Autodesk Inventor part; units mm, degrees
(part 2 of 2)
  arc A318 (-2.0424, 4.8628) -> (-1.7451, 4.6028) centre (-1.7451, 4.9028) ccw
  arc A319 (-4.2549, 4.6028) -> (-3.9576, 4.8628) centre (-4.2549, 4.9028) ccw
  line L244 (-4.5, 4.6028) -> (-4.2549, 4.6028)
  line L245 (-1.7451, 4.6028) -> (-1.5, 4.6028)
  arc A320 (-2.0424, 4.8628) -> (-2.4783, 5.8528) centre (-3.975, 4.6028) ccw
  line L246 (-3.5217, 5.8528) -> (-2.4783, 5.8528)
  arc A321 (-3.5217, 5.8528) -> (-3.9576, 4.8628) centre (-2.025, 4.6028) ccw
  arc A322 (-5.0424, 4.8628) -> (-4.7451, 4.6028) centre (-4.7451, 4.9028) ccw
  arc A323 (-7.2549, 4.6028) -> (-6.9576, 4.8628) centre (-7.2549, 4.9028) ccw
  line L247 (-7.5, 4.6028) -> (-7.2549, 4.6028)
  line L248 (-4.7451, 4.6028) -> (-4.5, 4.6028)
  arc A324 (-5.0424, 4.8628) -> (-5.4783, 5.8528) centre (-6.975, 4.6028) ccw
  line L249 (-6.5217, 5.8528) -> (-5.4783, 5.8528)
  arc A325 (-6.5217, 5.8528) -> (-6.9576, 4.8628) centre (-5.025, 4.6028) ccw
  arc A326 (24.9576, 4.8628) -> (25.2549, 4.6028) centre (25.2549, 4.9028) ccw
  arc A327 (22.7451, 4.6028) -> (23.0424, 4.8628) centre (22.7451, 4.9028) ccw
  line L250 (22.5, 4.6028) -> (22.7451, 4.6028)
  line L251 (25.2549, 4.6028) -> (25.5, 4.6028)
  arc A328 (24.9576, 4.8628) -> (24.5217, 5.8528) centre (23.025, 4.6028) ccw
  line L252 (23.4783, 5.8528) -> (24.5217, 5.8528)
  arc A329 (23.4783, 5.8528) -> (23.0424, 4.8628) centre (24.975, 4.6028) ccw
  arc A330 (21.9576, 4.8628) -> (22.2549, 4.6028) centre (22.2549, 4.9028) ccw
  arc A331 (19.7451, 4.6028) -> (20.0424, 4.8628) centre (19.7451, 4.9028) ccw
  line L253 (19.5, 4.6028) -> (19.7451, 4.6028)
  line L254 (22.2549, 4.6028) -> (22.5, 4.6028)
  arc A332 (21.9576, 4.8628) -> (21.5217, 5.8528) centre (20.025, 4.6028) ccw
  line L255 (20.4783, 5.8528) -> (21.5217, 5.8528)
  arc A333 (20.4783, 5.8528) -> (20.0424, 4.8628) centre (21.975, 4.6028) ccw
  arc A334 (18.9576, 4.8628) -> (19.2549, 4.6028) centre (19.2549, 4.9028) ccw
  arc A335 (16.7451, 4.6028) -> (17.0424, 4.8628) centre (16.7451, 4.9028) ccw
  line L256 (16.5, 4.6028) -> (16.7451, 4.6028)
  line L257 (19.2549, 4.6028) -> (19.5, 4.6028)
  arc A336 (18.9576, 4.8628) -> (18.5217, 5.8528) centre (17.025, 4.6028) ccw
  line L258 (17.4783, 5.8528) -> (18.5217, 5.8528)
  arc A337 (17.4783, 5.8528) -> (17.0424, 4.8628) centre (18.975, 4.6028) ccw
  arc A338 (15.9576, 4.8628) -> (16.2549, 4.6028) centre (16.2549, 4.9028) ccw
  arc A339 (13.7451, 4.6028) -> (14.0424, 4.8628) centre (13.7451, 4.9028) ccw
  line L259 (13.5, 4.6028) -> (13.7451, 4.6028)
  line L260 (16.2549, 4.6028) -> (16.5, 4.6028)
  arc A340 (15.9576, 4.8628) -> (15.5217, 5.8528) centre (14.025, 4.6028) ccw
  line L261 (14.4783, 5.8528) -> (15.5217, 5.8528)
  arc A341 (14.4783, 5.8528) -> (14.0424, 4.8628) centre (15.975, 4.6028) ccw
  arc A342 (12.9576, 4.8628) -> (13.2549, 4.6028) centre (13.2549, 4.9028) ccw
  arc A343 (10.7451, 4.6028) -> (11.0424, 4.8628) centre (10.7451, 4.9028) ccw
  line L262 (10.5, 4.6028) -> (10.7451, 4.6028)
  line L263 (13.2549, 4.6028) -> (13.5, 4.6028)
  arc A344 (12.9576, 4.8628) -> (12.5217, 5.8528) centre (11.025, 4.6028) ccw
  line L264 (11.4783, 5.8528) -> (12.5217, 5.8528)
  arc A345 (11.4783, 5.8528) -> (11.0424, 4.8628) centre (12.975, 4.6028) ccw
  arc A346 (9.9576, 4.8628) -> (10.2549, 4.6028) centre (10.2549, 4.9028) ccw
  arc A347 (7.7451, 4.6028) -> (8.0424, 4.8628) centre (7.7451, 4.9028) ccw
  line L265 (7.5, 4.6028) -> (7.7451, 4.6028)
  line L266 (10.2549, 4.6028) -> (10.5, 4.6028)
  arc A348 (9.9576, 4.8628) -> (9.5217, 5.8528) centre (8.025, 4.6028) ccw
  line L267 (8.4783, 5.8528) -> (9.5217, 5.8528)
  arc A349 (8.4783, 5.8528) -> (8.0424, 4.8628) centre (9.975, 4.6028) ccw
  arc A350 (6.9576, 4.8628) -> (7.2549, 4.6028) centre (7.2549, 4.9028) ccw
  arc A351 (4.7451, 4.6028) -> (5.0424, 4.8628) centre (4.7451, 4.9028) ccw
  line L268 (4.5, 4.6028) -> (4.7451, 4.6028)
  line L269 (7.2549, 4.6028) -> (7.5, 4.6028)
  arc A352 (6.9576, 4.8628) -> (6.5217, 5.8528) centre (5.025, 4.6028) ccw
  line L270 (5.4783, 5.8528) -> (6.5217, 5.8528)
  arc A353 (5.4783, 5.8528) -> (5.0424, 4.8628) centre (6.975, 4.6028) ccw
  arc A354 (3.9576, 4.8628) -> (4.2549, 4.6028) centre (4.2549, 4.9028) ccw
  arc A355 (1.7451, 4.6028) -> (2.0424, 4.8628) centre (1.7451, 4.9028) ccw
  line L271 (1.5, 4.6028) -> (1.7451, 4.6028)
  line L272 (4.2549, 4.6028) -> (4.5, 4.6028)
  arc A356 (3.9576, 4.8628) -> (3.5217, 5.8528) centre (2.025, 4.6028) ccw
  line L273 (2.4783, 5.8528) -> (3.5217, 5.8528)
  arc A357 (2.4783, 5.8528) -> (2.0424, 4.8628) centre (3.975, 4.6028) ccw
  arc A358 (0.9576, 4.8628) -> (1.2549, 4.6028) centre (1.2549, 4.9028) ccw
  arc A359 (-1.2549, 4.6028) -> (-0.9576, 4.8628) centre (-1.2549, 4.9028) ccw
  line L274 (-1.5, 4.6028) -> (-1.2549, 4.6028)
  line L275 (1.2549, 4.6028) -> (1.5, 4.6028)
  arc A360 (0.9576, 4.8628) -> (0.5217, 5.8528) centre (-0.975, 4.6028) ccw
  line L276 (-0.5217, 5.8528) -> (0.5217, 5.8528)
  arc A361 (-0.5217, 5.8528) -> (-0.9576, 4.8628) centre (0.975, 4.6028) ccw
  arc A362 (-2.0424, 4.8628) -> (-1.7451, 4.6028) centre (-1.7451, 4.9028) ccw
  arc A363 (-4.2549, 4.6028) -> (-3.9576, 4.8628) centre (-4.2549, 4.9028) ccw
  line L277 (-4.5, 4.6028) -> (-4.2549, 4.6028)
  line L278 (-1.7451, 4.6028) -> (-1.5, 4.6028)
  arc A364 (-2.0424, 4.8628) -> (-2.4783, 5.8528) centre (-3.975, 4.6028) ccw
  line L279 (-3.5217, 5.8528) -> (-2.4783, 5.8528)
  arc A365 (-3.5217, 5.8528) -> (-3.9576, 4.8628) centre (-2.025, 4.6028) ccw
  arc A366 (27.9576, 4.8628) -> (28.2549, 4.6028) centre (28.2549, 4.9028) ccw
  arc A367 (25.7451, 4.6028) -> (26.0424, 4.8628) centre (25.7451, 4.9028) ccw
  line L280 (25.5, 4.6028) -> (25.7451, 4.6028)
  line L281 (28.2549, 4.6028) -> (28.5, 4.6028)
  arc A368 (27.9576, 4.8628) -> (27.5217, 5.8528) centre (26.025, 4.6028) ccw
  line L282 (26.4783, 5.8528) -> (27.5217, 5.8528)
  arc A369 (26.4783, 5.8528) -> (26.0424, 4.8628) centre (27.975, 4.6028) ccw
  arc A370 (24.9576, 4.8628) -> (25.2549, 4.6028) centre (25.2549, 4.9028) ccw
  arc A371 (22.7451, 4.6028) -> (23.0424, 4.8628) centre (22.7451, 4.9028) ccw
  line L283 (22.5, 4.6028) -> (22.7451, 4.6028)
  line L284 (25.2549, 4.6028) -> (25.5, 4.6028)
  arc A372 (24.9576, 4.8628) -> (24.5217, 5.8528) centre (23.025, 4.6028) ccw
  line L285 (23.4783, 5.8528) -> (24.5217, 5.8528)
  arc A373 (23.4783, 5.8528) -> (23.0424, 4.8628) centre (24.975, 4.6028) ccw
  arc A374 (21.9576, 4.8628) -> (22.2549, 4.6028) centre (22.2549, 4.9028) ccw
  arc A375 (19.7451, 4.6028) -> (20.0424, 4.8628) centre (19.7451, 4.9028) ccw
  line L286 (19.5, 4.6028) -> (19.7451, 4.6028)
  line L287 (22.2549, 4.6028) -> (22.5, 4.6028)
  arc A376 (21.9576, 4.8628) -> (21.5217, 5.8528) centre (20.025, 4.6028) ccw
  line L288 (20.4783, 5.8528) -> (21.5217, 5.8528)
  arc A377 (20.4783, 5.8528) -> (20.0424, 4.8628) centre (21.975, 4.6028) ccw
  arc A378 (18.9576, 4.8628) -> (19.2549, 4.6028) centre (19.2549, 4.9028) ccw
  arc A379 (16.7451, 4.6028) -> (17.0424, 4.8628) centre (16.7451, 4.9028) ccw
  line L289 (16.5, 4.6028) -> (16.7451, 4.6028)
  line L290 (19.2549, 4.6028) -> (19.5, 4.6028)
  arc A380 (18.9576, 4.8628) -> (18.5217, 5.8528) centre (17.025, 4.6028) ccw
  line L291 (17.4783, 5.8528) -> (18.5217, 5.8528)
  arc A381 (17.4783, 5.8528) -> (17.0424, 4.8628) centre (18.975, 4.6028) ccw
  arc A382 (15.9576, 4.8628) -> (16.2549, 4.6028) centre (16.2549, 4.9028) ccw
  arc A383 (13.7451, 4.6028) -> (14.0424, 4.8628) centre (13.7451, 4.9028) ccw
  line L292 (13.5, 4.6028) -> (13.7451, 4.6028)
  line L293 (16.2549, 4.6028) -> (16.5, 4.6028)
  arc A384 (15.9576, 4.8628) -> (15.5217, 5.8528) centre (14.025, 4.6028) ccw
  line L294 (14.4783, 5.8528) -> (15.5217, 5.8528)
  arc A385 (14.4783, 5.8528) -> (14.0424, 4.8628) centre (15.975, 4.6028) ccw
  arc A386 (12.9576, 4.8628) -> (13.2549, 4.6028) centre (13.2549, 4.9028) ccw
  arc A387 (10.7451, 4.6028) -> (11.0424, 4.8628) centre (10.7451, 4.9028) ccw
  line L295 (10.5, 4.6028) -> (10.7451, 4.6028)
  line L296 (13.2549, 4.6028) -> (13.5, 4.6028)
  arc A388 (12.9576, 4.8628) -> (12.5217, 5.8528) centre (11.025, 4.6028) ccw
  line L297 (11.4783, 5.8528) -> (12.5217, 5.8528)
  arc A389 (11.4783, 5.8528) -> (11.0424, 4.8628) centre (12.975, 4.6028) ccw
  arc A390 (9.9576, 4.8628) -> (10.2549, 4.6028) centre (10.2549, 4.9028) ccw
  arc A391 (7.7451, 4.6028) -> (8.0424, 4.8628) centre (7.7451, 4.9028) ccw
  line L298 (7.5, 4.6028) -> (7.7451, 4.6028)
  line L299 (10.2549, 4.6028) -> (10.5, 4.6028)
  arc A392 (9.9576, 4.8628) -> (9.5217, 5.8528) centre (8.025, 4.6028) ccw
  line L300 (8.4783, 5.8528) -> (9.5217, 5.8528)
  arc A393 (8.4783, 5.8528) -> (8.0424, 4.8628) centre (9.975, 4.6028) ccw
  arc A394 (6.9576, 4.8628) -> (7.2549, 4.6028) centre (7.2549, 4.9028) ccw
  arc A395 (4.7451, 4.6028) -> (5.0424, 4.8628) centre (4.7451, 4.9028) ccw
  line L301 (4.5, 4.6028) -> (4.7451, 4.6028)
  line L302 (7.2549, 4.6028) -> (7.5, 4.6028)
  arc A396 (6.9576, 4.8628) -> (6.5217, 5.8528) centre (5.025, 4.6028) ccw
  line L303 (5.4783, 5.8528) -> (6.5217, 5.8528)
  arc A397 (5.4783, 5.8528) -> (5.0424, 4.8628) centre (6.975, 4.6028) ccw
  arc A398 (3.9576, 4.8628) -> (4.2549, 4.6028) centre (4.2549, 4.9028) ccw
  arc A399 (1.7451, 4.6028) -> (2.0424, 4.8628) centre (1.7451, 4.9028) ccw
  line L304 (1.5, 4.6028) -> (1.7451, 4.6028)
  line L305 (4.2549, 4.6028) -> (4.5, 4.6028)
  arc A400 (3.9576, 4.8628) -> (3.5217, 5.8528) centre (2.025, 4.6028) ccw
  line L306 (2.4783, 5.8528) -> (3.5217, 5.8528)
  arc A401 (2.4783, 5.8528) -> (2.0424, 4.8628) centre (3.975, 4.6028) ccw
  arc A402 (0.9576, 4.8628) -> (1.2549, 4.6028) centre (1.2549, 4.9028) ccw
  arc A403 (-1.2549, 4.6028) -> (-0.9576, 4.8628) centre (-1.2549, 4.9028) ccw
  line L307 (-1.5, 4.6028) -> (-1.2549, 4.6028)
  line L308 (1.2549, 4.6028) -> (1.5, 4.6028)
  arc A404 (0.9576, 4.8628) -> (0.5217, 5.8528) centre (-0.975, 4.6028) ccw
  line L309 (-0.5217, 5.8528) -> (0.5217, 5.8528)
  arc A405 (-0.5217, 5.8528) -> (-0.9576, 4.8628) centre (0.975, 4.6028) ccw
  point P0 (0, -10)
  point P1 (0, 0)
  point P2 (-0.5217, 5.8528)
  point P3 (-25, 5.8528)
  point P4 (25, 5.8528)
  point P5 (25, 4.7446)
  point P6 (-25, 4.7446)
  dimension "d6" = 16.2338
  dimension "d8" = 100
  dimension "d9" = 0.419
  dimension "d10" = 0.8
  dimension "d12" = 0.3
  dimension "d13" = 0.525
  dimension "d14" = 0.3
  dimension "d15" = 1.95
  dimension "d16" = 2.475
  dimension "d17" = 0.9783
  dimension "d19" = 1.0433
  dimension "d21" = 10
  dimension "d22" = 0.2451
  dimension "d23" = 0.2451
  dimension "d24" = 0.3
  dimension "d25" = 2.7549
  dimension "d26" = 1.25
  dimension "d29" = 0.5217
  dimension "d54" = 3
  dimension "d57" = 3
  constraints: 812 point on circle, 616 end point, 406 centre point, 6 horizontal alignment, 5 tangent, 3 horizontal, 3 parallel, 1 midpoint, 1 point on line, 1 vertical alignment, 1887 other
  measures "d6" radius of A0
  measures "d8" distance of L0.start L0.end
  measures "d9" radial gap between concentric circles of A3 A0
  measures "d10" radial gap between concentric circles of A3 A5
  measures "d12" distance from line of L7 A6.centre
  measures "d13" distance of L7.start A8.centre
  measures "d14" radius of A6
  measures "d15" radius of A7
  measures "d16" distance of L7.start A7.centre
  measures "d17" horizontal distance of L7.start L8.start
  measures "d19" distance of L8.start L8.end
  measures "d21" distance of point (0, 0) point (0, -10)
  measures "d22" distance of L7.start L7.end
  measures "d23" distance of L9.start L9.end
  measures "d24" radius of A9
  measures "d25" distance of L7.start L9.start
  measures "d26" distance from line of L7.start L8
  measures "d29" horizontal distance of point (0, 0) L8.end
  measures "d54" distance of A8.start A10.start
  measures "d57" distance of A8.start A46.start
extrude "押し出し2" cut sketch "スケッチ2" against normal through all contours L10 L11 L12 L3 | L3 L12 A326 A328 L252 A329 A327 L250 L221 A286 A288 L222 A289 A287 L220 L191 A246 A248 L192 A249 A247 L190 L161 A206 A208 L162 A209 A207 L160 L131 A166 A168 L132 A169 A167 L130 L101 A126 A128 L102 A129 A127 L100 L71 A86 A88 L72 A89 A87 L70 L41 A46 A48 L42 A49 A47 L40 L9 A9 A8 L8 A7 A6 L7 L14 A10 A12 L15 A13 A11 L13 L17 A14 A16 L18 A17 A15 L16 L20 A18 A20 L21 A21 A19 L19 L23 A22 A24 L24 A25 A23 L22 L26 A26 A28 L27 A29 A27 L25 L29 A30 A32 L30 A33 A31 L28 L32 A34 A36 L33 A37 A35 L31 L35 A38 A40 L36 A41 A39 L10
sketch "スケッチ6" plane through (0, 0, 8) normal (0, 0, 1) x (1, 0, 0)
  line L0 (-25, -9) -> (25, -9) projected
  line L1 (-25, 4.7446) -> (-25, -9) projected
  line L2 (-25, -9) -> (25, -9)
  line L3 (25, -9) -> (25, 6.6528)
  line L4 (25, 6.6528) -> (-25, 6.6528)
  line L5 (-25, 6.6528) -> (-25, -9)
  line L6 (-23.4783, 5.8528) -> (-24.5217, 5.8528) projected
  point P0 (0, 0)
  dimension "d61" = 0.8
  constraints: 8 end point, 2 parallel, 1 horizontal, 1 perpendicular, 1 vertical alignment
  measures "d61" distance between parallel lines of L4 L6
extrude "押し出し4" add sketch "スケッチ6" along normal blind 8
sketch "スケッチ3" plane through (0, 0, 0) normal (0, 0, 1) x (1, 0, 0)
  point P0 (0, 0)
  point P1 (-15, 0)
  point P2 (15, 0)
  dimension "d40" = 15
  dimension "d41" = 15
  constraints: 2 horizontal alignment
  measures "d40" distance of point (0, 0) point (-15, 0)
  measures "d41" distance of point (15, 0) point (0, 0)
hole "穴1" at (-15, 0, 0) at (15, 0, 0) direction (0, 0, 1) diameter 4.3 end through all clearance for "Socket Head Cap Screw" size "M4" standard "Ansi Metric M Profile"
equation "\"d23\" = d22"
equation "\"d29\" = 0.5 * d19"
